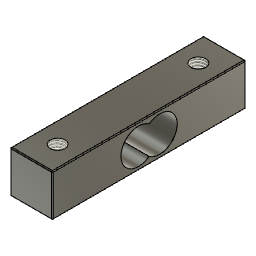
GYARB_Vikt sensor (Autodesk Fusion 360 design; units mm, degrees)
Autodesk Fusion 360 part; units mm, degrees
sketch "Sketch1" plane through (0, 0, 0) normal (1, 0, 0) x (0, 1, 0)
  line L0 (-27.5, 6) -> (27.5, 6)
  line L1 (27.5, 6) -> (27.5, -6)
  line L2 (27.5, -6) -> (-27.5, -6)
  line L3 (-27.5, -6) -> (-27.5, 6)
  line L4 (-27.5, 6) -> (27.5, -6) construction
  line L5 (27.5, 6) -> (-27.5, -6) construction
  line L6 (0, 0) -> (-3, 0) construction
  circle A0 centre (-3, 0) radius 5
  line L7 (0, 0) -> (3, 0) construction
  circle A1 centre (3, 0) radius 5
  dimension "d65" = 55
  dimension "d66" = 12
  dimension "d67" = 3
  dimension "d68" = 3
  dimension "d69" = 10
  constraint horizontal L0
  constraint perpendicular L0 L1
  constraint parallel L0 L2
  constraint parallel L1 L3
  constraint coincident L4 L6.start
  constraint coincident L5 L6.start
  constraint coincident L6.start L7.start
  constraint parallel L0 L6
  constraint coincident L6.end A0.centre
  constraint horizontal L7
  constraint coincident L7.end A1.centre
  measures "d65" distance of L1.end L2.end
  measures "d66" distance of L0.end L1.end
  measures "d67" distance of L6.start L6.end
  measures "d68" distance of L6.start L7.end
  measures "d69" diameter of A1
extrude "Extrude1" add sketch "Sketch1" along normal blind 12
move_body "Move1" bodies 1 to x (1, 0, 0) y (0, 1, 0) z (0, 0, 1) at (-5, 0, 0)
move_body "Move2" bodies 1 to x (1, 0, 0) y (0, 1, 0) z (0, 0, 1) at (-1, 0, 0)
sketch "Sketch2" plane through (0, 0, 6) normal (0, 0, 1) x (-1, 0, 0)
  line L0 (6, -27.5) -> (6, 27.5)
  line L1 (6, 27.5) -> (-6, 27.5)
  line L2 (-6, 27.5) -> (-6, -27.5)
  line L3 (-6, -27.5) -> (6, -27.5)
  line L4 (0, 27.5) -> (0, 20) construction
  circle A0 centre (0, 20) radius 2.5
  line L5 (0, -27.5) -> (0, -20) construction
  circle A1 centre (0, -20) radius 2.5
  dimension "d72" = 7.5
  dimension "d73" = 5
  dimension "d74" = 5
  constraint midpoint L1 L4.start
  constraint perpendicular L1 L4
  constraint coincident L4.end A0.centre
  constraint midpoint L3 L5.start
  constraint perpendicular L3 L5
  constraint coincident L5.end A1.centre
  measures "d72" distance of L4.start L4.end
  measures "d73" diameter of A0
  measures "d74" diameter of A1
hole "Hole1" at (0, -20, 6) at (0, 20, 6) direction (0, 0, -1) diameter 4.234 depth 40 tip angle 118
thread "Thread1" "ISO Metric profile 5.0 M5x0.8 6H"
fillet "Fillet1" radius 0.25 12 edges at (6, 0, 6) (0, 27.5, 6) (6, 27.5, 0) (-6, 27.5, 0) (0, 27.5, -6) (6, 0, -6) (-6, 0, -6) (-6, 0, 6) (0, -27.5, 6) (6, -27.5, 0) (0, -27.5, -6) (-6, -27.5, 0)
move_body "Move3" bodies 1 to x (1, 0, 0) y (0, 1, 0) z (0, 0, 1) at (0, 145, 230)
